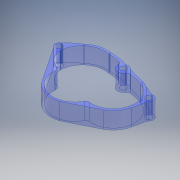
# Autodesk Inventor part: body gauche
Saved by Autodesk Inventor 2018.1 (Build 221171000, 171)
## iProperties
Created: 2022-07-20
Part Number: body gauche
Material: Generic
Document SubType Name: Modeling
Designer: mouta
Density: 1 g/cm^3
Appearance: Default
Author: mouta
Autodesk Inventor part; units mm, degrees
ref_plane "YZ Plane" through (0, 0, 0) normal (1, 0, 0) x (0, 1, 0)
ref_plane "XZ Plane" through (0, 0, 0) normal (0, 1, 0) x (-1, 0, 0)
ref_plane "XY Plane" through (0, 0, 0) normal (0, 0, 1) x (1, 0, 0)
sketch "Sketch1" plane through (0, 0, 0) normal (0, 0, 1) x (1, 0, 0)
  circle A0 centre (0, 0) radius 5
  circle A1 centre (149.4, 0) radius 5
  circle A2 centre (85.7991, 21.6971) radius 5
  circle A3 centre (110.2989, -19.8991) radius 12.5
  arc A4 (154.885, -2.4321) -> (154.9491, -2.282) centre (149.4, 0) ccw
  line L0 (-1.9594, 5.6711) -> (-0.9713, 5.9209)
  line L1 (94.051, 25.713) -> (120.8026, 18.6971)
  arc A5 (131.5219, 14.0064) -> (120.0887, 18.8843) centre (110.2989, -19.8991) ccw
  line L2 (0, 0) -> (4.8474, 1.2258)
  line L3 (80.8741, 20.8344) -> (85.7991, 21.6971)
  arc A6 (125.9738, -56.7) -> (149.4311, -28.1861) centre (110.2989, -19.8991) ccw
  line L4 (80.7723, -79.2884) -> (129.3991, -55.0443)
  line L5 (-2.1405, -7.4309) -> (37.9799, -67.1663)
  arc A7 (90.3858, 23.6876) -> (86.8225, 21.8764) centre (110.2989, -19.8991) ccw
  arc A8 (33.9775, -61.2072) -> (80.7723, -79.2884) centre (68.0362, -42.6558) ccw
  arc A9 (-3.2331, 6.2086) -> (-3.6699, -5.9609) centre (0, 0) ccw
  line L6 (131.5219, 14.0064) -> (145.3135, 8.2114)
  line L7 (150.7621, 5.922) -> (151.3594, 5.6711)
  line L8 (154.928, -2.2287) -> (154.885, -2.4321)
  line L9 (153.6652, -8.1921) -> (149.4311, -28.1861)
  arc A10 (154.9491, -2.282) -> (154.3356, -0.8001) centre (110.2989, -19.8991) ccw
  arc A11 (151.6581, 4.4611) -> (150.7621, 5.922) centre (110.2989, -19.8991) ccw
  arc A12 (-0.9713, 5.9209) -> (-1.9594, 5.6711) centre (0, 0) ccw
  arc A13 (-4.6746, 3.7614) -> (-4.9033, 3.458) centre (55.8634, -42.1071) ccw
  arc A14 (-4.6746, 3.7614) -> (-4.9033, 3.458) centre (0, 0) ccw
  arc A15 (-3.2331, 6.2086) -> (-1.7498, 7.3852) centre (-5.5425, 10.6433) ccw
  arc A16 (-2.1405, -7.4309) -> (-3.6699, -5.9609) centre (-6.2912, -10.2187) ccw
  arc A17 (50.3563, 33.7779) -> (18.6552, 24.2587) centre (44.1835, -3.2106) ccw
  arc A18 (80.9569, 29.5804) -> (51.4686, 33.7181) centre (55.8634, -42.1071) ccw
  arc A19 (17.7599, 23.5959) -> (-1.7498, 7.3852) centre (55.8634, -42.1071) ccw
  arc A20 (17.7599, 23.5959) -> (18.6552, 24.2587) centre (15.2515, 27.9212) ccw
  arc A21 (50.3563, 33.7779) -> (51.4686, 33.7181) centre (51.1793, 38.7097) ccw
  arc A22 (91.6578, 27.1447) -> (83.8358, 29.4525) centre (85.7991, 21.6971) ccw
  arc A23 (155.0349, -5.6787) -> (148.0771, 7.8899) centre (149.4, 0) ccw
  arc A24 (155.0349, -5.6787) -> (153.6652, -8.1921) centre (158.5567, -9.2279) ccw
  arc A25 (145.3135, 8.2114) -> (148.0771, 7.8899) centre (147.2503, 12.821) ccw
  arc A26 (80.9569, 29.5804) -> (83.8358, 29.4525) centre (82.6088, 34.2996) ccw
  arc A27 (91.6578, 27.1447) -> (94.051, 25.713) centre (95.3194, 30.5494) ccw
  point P0 (90.8386, 26.5555)
  point P1 (111.3369, -59.8857)
  point P2 (-4.37, -4.1113)
  point P3 (148.3758, 6.9247)
  point P4 (154.3524, -4.9471)
  point P5 (-2.8318, -6.4017)
  point P6 (92.4582, 26.1307)
  point P7 (146.8277, 7.5752)
  point P8 (154.0164, -6.5337)
  dimension "d3" = 10
  dimension "d5" = 10
  dimension "d15" = 10
  dimension "d18" = 25
  dimension "d20" = 12
  dimension "d88" = 14
  dimension "d104" = 75
  dimension "d105" = 5
  dimension "d112" = 16
  dimension "d113" = 16
  dimension "d114" = 5
  constraints: 61 point on circle, 27 centre point, 20 end point, 17 tangent, 10 point on line, 6 coincident, 4 equal radius, 3 other
  measures "d5" diameter of A1
  measures "d15" diameter of A2
  measures "d18" diameter of A3
  measures "d20" diameter of A4
  measures "d88" diameter of A9
  measures "d104" diameter of A17
  measures "d105" radius of A20
  measures "d112" diameter of A22
  measures "d113" diameter of A23
  measures "d114" radius of A24
extrude "Extrusion2" add sketch "Sketch1" along normal blind 28 contours L8 A10 A4 | L1 A5 L6 A25 A23 A24 L9 A6 L4 A8 L5 A16 A9 A15 A19 A20 A17 A21 A18 A26 A22 A27 | A13 A14
sketch "Sketch13" plane through (0, 0, 28) normal (0, 0, 1) x (1, 0, 0)
  arc A0 (105.7808, -55.6145) -> (122.4659, 13.9825) centre (110.2989, -19.8991) ccw
  line L0 (32.2727, -40.0871) -> (32.3131, -38.891)
  circle A1 centre (85.7991, 21.6971) radius 5 projected
  arc A2 (122.3009, 14.0385) -> (99.574, 19.2733) centre (79.666, -119.1093) ccw
  arc A3 (75.8397, 22.5968) -> (71.8542, 27.9468) centre (70.8599, 23.0467) ccw
  arc A4 (99.574, 19.2733) -> (94.5077, 16.7819) centre (98.8621, 14.3243) ccw
  arc A5 (105.7808, -55.6145) -> (100.6423, -58.4183) centre (105.1533, -60.575) ccw
  arc A6 (32.3131, -38.891) -> (31.6808, -35.0382) centre (22.3188, -38.553) ccw
  arc A7 (71.8542, 27.9468) -> (53.5851, 30.0522) centre (55.1602, -36.5967) ccw
  arc A8 (45.4586, 29.4346) -> (46.2799, 29.4767) centre (45.6139, 34.4322) ccw
  arc A9 (122.4659, 13.9825) -> (122.3009, 14.0385) centre (120.7761, 9.2767) ccw
  arc A10 (32.2727, -40.0871) -> (100.6423, -58.4183) centre (68.36, -42.1569) ccw
  arc A11 (75.8397, 22.5968) -> (94.5077, 16.7819) centre (85.7991, 21.6971) ccw
  arc A12 (21.1272, 20.7085) -> (21.4488, 20.9624) centre (18.1914, 24.7558) ccw
  arc A13 (52.3778, 30.1709) -> (7.5869, -5.4513) centre (44.3656, -5.7255) ccw
  arc A14 (7.6133, -6.0028) -> (28.5671, -32.0476) centre (38.2081, -2.8397) ccw
  arc A15 (26.215, -29.3432) -> (26.5512, -29.4928) centre (38.2081, -2.8397) ccw
  arc A16 (52.3778, 30.1709) -> (53.5851, 30.0522) centre (53.467, 35.0508) ccw
  arc A17 (7.5869, -5.4513) -> (7.6133, -6.0028) centre (12.5868, -5.4886) ccw
  arc A18 (31.6808, -35.0382) -> (28.5671, -32.0476) centre (26.9998, -36.7956) ccw
  point P0 (0, 0)
  point P1 (44.2138, -2.45)
  point P2 (68.1634, -42.8903)
  point P3 (32.5739, -31.1818)
  dimension "d97" = 5
  dimension "d99" = 10
  dimension "d106" = 5
  dimension "d107" = 5
  dimension "d108" = 5
  dimension "d111" = 5
  constraints: 37 point on circle, 18 centre point, 14 tangent, 4 equal radius, 2 coincident, 2 end point, 1 point on line
  measures "d97" radius of A3
  measures "d99" radius of A6
  measures "d106" radius of A8
  measures "d107" radius of A9
  measures "d108" radius of A12
  measures "d111" radius of A16
extrude "Extrusion18" cut sketch "Sketch13" against normal blind 30 contours A5 A10 L0 A6 A18 A14 A17 A13 A16 A7 A3 A11 A4 A2 A9 A0
body "Solid2"
